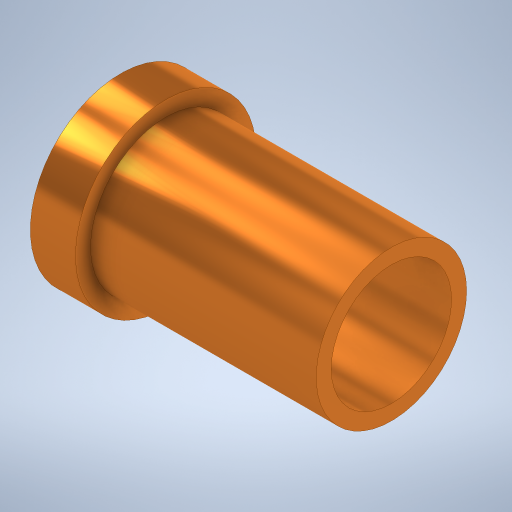
# Autodesk Inventor part: SechDurchmesser_ring
Saved by Autodesk Inventor 2024 (Build 280153000, 153)
## iProperties
Created: 2024-03-07
Part Number: SechDurchmesser_ring
Material: Gold
Document SubType Name: Modeling
Designer: ffogue
Density: 19.3 g/cm^3
Appearance: Metall - 1600F (heiß)
Author: ffogue
Autodesk Inventor part; units mm, degrees
ref_plane "YZ Plane" through (0, 0, 0) normal (1, 0, 0) x (0, 1, 0)
ref_plane "XZ Plane" through (0, 0, 0) normal (0, 1, 0) x (-1, 0, 0)
ref_plane "XY Plane" through (0, 0, 0) normal (0, 0, 1) x (1, 0, 0)
sketch "Skizze1" plane through (0, 0, 0) normal (0, 0, 1) x (1, 0, 0)
  line L0 (0, 0) -> (9, 0)
  line L1 (0, 0) -> (0, 3)
  line L2 (0, 3) -> (1.5, 3)
  line L3 (1.5, 3) -> (1.5, 2.5)
  line L4 (1.5, 2.5) -> (9, 2.5)
  line L5 (9, 2.5) -> (9, 0)
  point P0 (1.5, 2.75)
  dimension "d0" = 1.5
  dimension "d1" = 6
  dimension "d2" = 5
  dimension "d3" = 9
  constraints: 12 end point, 4 perpendicular, 2 coincident, 1 horizontal, 1 midpoint, 1 point on line, 1 vertical
  measures "d0" distance from line of point (1.5, 2.75) L1
  measures "d1" diameter of L2 L0
  measures "d2" diameter of L4 L0
  measures "d3" distance between parallel lines of L5 L1
revolve "Umdrehung1" add sketch "Skizze1" angle 360 about axis through (0, 0, 0) along (1, 0, 0)
sketch "Skizze2" plane through (9, 0, 0) normal (1, 0, 0) x (0, 0, -1)
  circle A0 centre (0, 0) radius 2.5 projected
  constraints: 1 coincident
hole "Bohrung1" at (9, 0, 0) direction (-1, 0, 0) diameter 4 end through all
